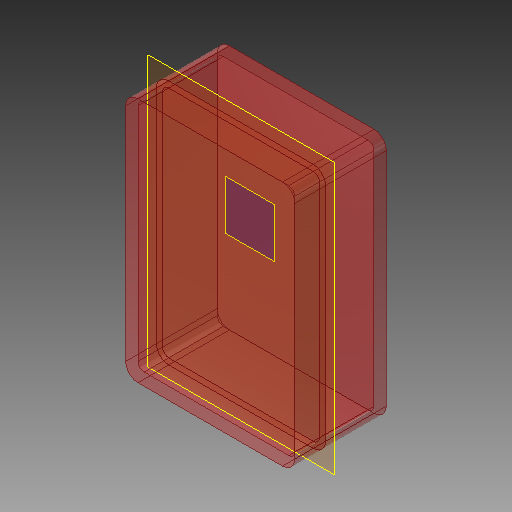
# Autodesk Inventor part: bottom
Saved by Autodesk Inventor 2020 (Build 240168000, 168)
## iProperties
Created: 2019-03-25
Part Number: bottom
Material: Generic
Document SubType Name: Modeling
Designer: erwin
Density: 1 g/cm^3
Appearance: Default
Author: erwin
Autodesk Inventor part; units mm, degrees
ref_plane "YZ Plane" through (0, 0, 0) normal (1, 0, 0) x (0, 1, 0)
ref_plane "XZ Plane" through (0, 0, 0) normal (0, 1, 0) x (-1, 0, 0)
ref_plane "Work Plane3" through (-33.721, -16.0631, -8.3772) normal (0, 0, -1) x (-1, 0, 0)
sketch "Sketch2" plane through (-33.721, -16.0631, -8.3772) normal (0, 0, -1) x (-1, 0, 0)
  line L0 (3.351, 52.725) -> (-51.649, 52.725)
  line L1 (-51.649, 52.725) -> (-51.649, -27.275)
  line L2 (-51.649, -27.275) -> (3.351, -27.275)
  line L3 (3.351, -27.275) -> (3.351, 52.725)
  line L4 (3.351, 52.725) -> (-51.649, -27.275) construction
  line L5 (-51.649, 52.725) -> (3.351, -27.275) construction
  line L6 (-25.524, -24.775) -> (-3.524, -24.775) projected
  line L7 (-0.024, 32.975) -> (-0.024, 14.6) projected
  line L8 (-48.274, -10.275) -> (-48.274, 32.975) projected
  line L9 (-3.524, 50.225) -> (-25.524, 50.225) projected
  point P0 (-33.721, 16.0631)
  point P1 (-24.149, 12.725)
  dimension "d2" = 55
  dimension "d3" = 80
  dimension "d4" = 2.5
  dimension "d5" = 3.375
  dimension "d6" = 3.375
  dimension "d7" = 2.5
  constraints: 12 end point, 2 midpoint, 2 parallel, 1 horizontal, 1 perpendicular
  measures "d2" distance of L2.end L1.end
  measures "d3" distance of L1.end L0.end
  measures "d4" distance between parallel lines of L0 L9
  measures "d5" distance between parallel lines of L3 L7
  measures "d6" distance between parallel lines of L1 L8
  measures "d7" distance between parallel lines of L2 L6
ref_plane "Work Plane4" through (-28.697, -42.3381, 21.3728) normal (0, 0, 1) x (1, 0, 0)
extrude "Extrusion1" add sketch "Sketch2" against normal up to surface (29.75 mm away)
fillet "Fillet1" radius 4 4 edges at (-37.072, -43.3381, 6.4978) (17.928, -43.3381, 6.4978) (17.928, 36.6619, 6.4978) (-37.072, 36.6619, 6.4978)
shell "Shell1" thickness 2 removed faces 0
ref_plane "Work Plane5" through (-8.197, -40.8381, 11.3728) normal (0, 0, 1) x (1, 0, 0)
split body "Split1" result two bodies by plane through (-8.197, -40.8381, 11.3728) normal (0, 0, 1) first body at (-18.7387, 8.6619, 20.8728)
equation "\"d6\" = d5"
equation "\"d7\" = d4"
body "Solid2"
body "Solid3"
